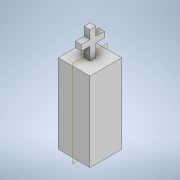
# Autodesk Inventor part: tiered-king
Saved by Autodesk Inventor 2021 (Build 250183000, 183)
## iProperties
Created: 2021-01-20
Part Number: tiered-king
Material: Generic
Document SubType Name: Modeling
Designer: Luke Kamols
Density: 1 g/cm^3
Appearance: Default
Author: Luke Kamols
Autodesk Inventor part; units mm, degrees
ref_plane "YZ Plane" through (0, 0, 0) normal (1, 0, 0) x (0, 1, 0)
ref_plane "XZ Plane" through (0, 0, 0) normal (0, 1, 0) x (-1, 0, 0)
ref_plane "XY Plane" through (0, 0, 0) normal (0, 0, 1) x (1, 0, 0)
sketch "Sketch1" plane through (0, 0, 0) normal (0, 1, 0) x (-1, 0, 0)
  line L0 (0, 0) -> (22, 0)
  line L1 (22, 0) -> (22, -22)
  line L2 (22, -22) -> (0, -22)
  line L3 (0, -22) -> (0, 0)
  dimension "d0" = 22
  dimension "d1" = 22
  constraints: 8 end point, 2 parallel, 1 horizontal, 1 perpendicular
  measures "d0" distance of L1.end L2.end
  measures "d1" distance of L0.end L1.end
extrude "Extrusion1" add sketch "Sketch1" along normal blind 55
ref_plane "Work Plane1" through (-11, 0, 0) normal (1, 0, 0) x (0, 0, -1)
sketch "Sketch2" plane through (-11, 0, 0) normal (1, 0, 0) x (0, 0, -1)
  line L0 (0, 55) -> (22, 55) projected
  line L1 (11, 55) -> (9, 55)
  line L2 (22, 55) -> (0, 55) projected
  line L3 (9, 55) -> (9, 64)
  line L4 (9, 64) -> (3, 64)
  line L5 (3, 64) -> (3, 68)
  line L6 (3, 68) -> (9, 68)
  line L7 (9, 68) -> (9, 74)
  line L8 (9, 74) -> (13, 74)
  line L9 (13, 74) -> (13, 68)
  line L10 (13, 68) -> (19, 68)
  line L11 (19, 68) -> (19, 64)
  line L12 (19, 64) -> (13, 64)
  line L13 (13, 64) -> (13, 55)
  point P0 (0, 0)
  dimension "d4" = 2
  dimension "d5" = 9
  dimension "d6" = 6
  dimension "d7" = 4
  dimension "d8" = 6
  dimension "d9" = 4
  dimension "d10" = 6
  constraints: 24 end point, 8 perpendicular, 4 point on line, 1 horizontal, 1 midpoint, 1 vertical
  measures "d4" distance of L1.start L1.end
  measures "d5" distance of L1.end L3.end
  measures "d6" distance of L3.end L4.end
  measures "d7" distance of L4.end L5.end
  measures "d8" distance of L6.end L7.end
  measures "d9" distance of L7.end L8.end
  measures "d10" distance of L9.end L10.end
extrude "Extrusion2" add sketch "Sketch2" along normal mid plane 4
body "Solid1"
